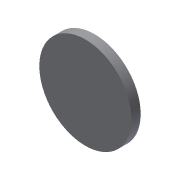
# Autodesk Inventor part: 00_Mirror_10mmDia
Saved by Autodesk Inventor 2019 (Build 230136000, 136)
## iProperties
Created: 2019-10-10
Part Number: 00_Mirror_10mmDia
Material: Generic
Document SubType Name: Modeling
Designer: diederichbenedict
Density: 1 g/cm^3
Appearance: Default
Author: diederichbenedict
Autodesk Inventor part; units mm, degrees
ref_plane "YZ Plane" through (0, 0, 0) normal (1, 0, 0) x (0, 1, 0)
ref_plane "XZ Plane" through (0, 0, 0) normal (0, 1, 0) x (-1, 0, 0)
ref_plane "XY Plane" through (0, 0, 0) normal (0, 0, 1) x (1, 0, 0)
sketch "Sketch1" plane through (0, 0, 0) normal (0, 0, 1) x (1, 0, 0)
  ellipse E0 centre (24.2654, -26.1396) end of major axis (22.8349, -26.1396) minor radius 1.0115 (25.6959, -26.1396) -> (22.8349, -26.1396) ccw projected
  line L0 (22.8349, -26.1396) -> (25.6959, -26.1396) projected
  circle A0 centre (24.2654, -26.1396) radius 5
  dimension "d3" = 10
  constraints: 1 centre point, 1 coincident, 1 other
  measures "d3" diameter of A0
extrude "Extrusion1" add sketch "Sketch1" along normal blind 1 contours L0 E0 | A0
body "Solid1"
